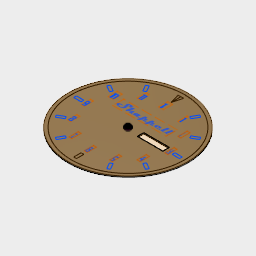
Dial (Autodesk Fusion 360 design; units mm, degrees)
Autodesk Fusion 360 part; units mm, degrees
sketch "Sketch4" plane through (0, 0, 0) normal (0, 1, 0) x (1, 0, 0)
  circle A0 centre (0, 0) radius 16.375
  dimension "d2" = 32.75
  measures "d2" diameter of A0
extrude "Extrude1" add sketch "Sketch4" along normal blind 0.35
sketch "Sketch5" plane through (0, 0.35, 0) normal (0, 1, 0) x (-1, 0, 0)
  circle A0 centre (0, 0) radius 16.375
  circle A1 centre (0, 0) radius 0.85
  line L0 (-3.45, -0.875) -> (-10.45, -0.875)
  line L1 (-10.45, -0.875) -> (-10.45, 0.875)
  line L2 (-10.45, 0.875) -> (-3.45, 0.875)
  line L3 (-3.45, 0.875) -> (-3.45, -0.875)
  dimension "d11" = 1.7
  dimension "d12" = 7
  dimension "d14" = 1.75
  dimension "d15" = 3.45
  dimension "d16" = 0.875
  measures "d11" diameter of A1
  measures "d12" distance of L0.start L0.end
  measures "d14" distance of L0.end L1.end
  measures "d15" distance of A0.centre L3
  measures "d16" distance of A0.centre L0.start
extrude "Extrude2" cut sketch "Sketch5" against normal through all contours A1 | L0 L1 L2 L3
sketch "Sketch7" plane through (0, 0.35, 0) normal (0, 1, 0) x (-1, 0, 0)
  circle A0 centre (0, 0) radius 0.85
  line L0 (-3.45, 0.875) -> (-3.45, -0.875)
  line L1 (-3.45, -0.875) -> (-10.45, -0.875)
  line L2 (-10.45, -0.875) -> (-10.45, 0.875)
  line L3 (-10.45, 0.875) -> (-3.45, 0.875)
  circle A1 centre (0, 0) radius 16.375
  line L4 (0.375, 12.5) -> (-0.375, 12.5)
  line L5 (-0.375, 12.5) -> (-0.375, 14.5)
  line L6 (-0.375, 14.5) -> (0.375, 14.5)
  line L7 (0.375, 14.5) -> (0.375, 12.5)
  circle A2 centre (0, 0) radius 15.5
  line L8 (-6.5748, 10.6378) -> (-7.5748, 12.3699)
  line L9 (-6.9252, 12.7449) -> (-5.9252, 11.0128)
  line L10 (-5.9252, 11.0128) -> (-6.5748, 10.6378)
  line L11 (-7.5748, 12.3699) -> (-6.9252, 12.7449)
  line L12 (-11.0128, 5.9252) -> (-12.7449, 6.9252)
  line L13 (-12.3699, 7.5748) -> (-10.6378, 6.5748)
  line L14 (-10.6378, 6.5748) -> (-11.0128, 5.9252)
  line L15 (-12.7449, 6.9252) -> (-12.3699, 7.5748)
  line L16 (-10.6378, -6.5748) -> (-12.3699, -7.5748)
  line L17 (-12.7449, -6.9252) -> (-11.0128, -5.9252)
  line L18 (-11.0128, -5.9252) -> (-10.6378, -6.5748)
  line L19 (-12.3699, -7.5748) -> (-12.7449, -6.9252)
  line L20 (-5.9252, -11.0128) -> (-6.9252, -12.7449)
  line L21 (-7.5748, -12.3699) -> (-6.5748, -10.6378)
  line L22 (-6.5748, -10.6378) -> (-5.9252, -11.0128)
  line L23 (-6.9252, -12.7449) -> (-7.5748, -12.3699)
  line L24 (6.5748, -10.6378) -> (7.5748, -12.3699)
  line L25 (6.9252, -12.7449) -> (5.9252, -11.0128)
  line L26 (5.9252, -11.0128) -> (6.5748, -10.6378)
  line L27 (7.5748, -12.3699) -> (6.9252, -12.7449)
  line L28 (11.0128, -5.9252) -> (12.7449, -6.9252)
  line L29 (12.3699, -7.5748) -> (10.6378, -6.5748)
  line L30 (10.6378, -6.5748) -> (11.0128, -5.9252)
  line L31 (12.7449, -6.9252) -> (12.3699, -7.5748)
  line L32 (10.6378, 6.5748) -> (12.3699, 7.5748)
  line L33 (12.7449, 6.9252) -> (11.0128, 5.9252)
  line L34 (11.0128, 5.9252) -> (10.6378, 6.5748)
  line L35 (12.3699, 7.5748) -> (12.7449, 6.9252)
  line L36 (5.9252, 11.0128) -> (6.9252, 12.7449)
  line L37 (7.5748, 12.3699) -> (6.5748, 10.6378)
  line L38 (6.5748, 10.6378) -> (5.9252, 11.0128)
  line L39 (6.9252, 12.7449) -> (7.5748, 12.3699)
  line L40 (0.75, -14.5) -> (-0.75, -14.5)
  line L41 (-0.75, -14.5) -> (0, -11.75)
  line L42 (0, -11.75) -> (0.75, -14.5)
  line L43 (0, -14.5) -> (0, -11.75)
  line L44 (-12.5, -0.375) -> (-14.5, -0.375)
  line L45 (-14.5, 0.375) -> (-12.5, 0.375)
  line L46 (-12.5, 0.375) -> (-12.5, -0.375)
  line L47 (-14.5, -0.375) -> (-14.5, 0.375)
  line L48 (12.5, 0.375) -> (14.5, 0.375)
  line L49 (14.5, -0.375) -> (12.5, -0.375)
  line L50 (12.5, -0.375) -> (12.5, 0.375)
  line L51 (14.5, 0.375) -> (14.5, -0.375)
  dimension "d20" = 0.75
  dimension "d21" = 2
  dimension "d24" = 31
  dimension "d26" = 0.375
  dimension "d31" = 2.75
  dimension "d32" = 1.5
  dimension "d33" = 0.75
  dimension "d34" = 14.5
  dimension "d35" = 14.5
  measures "d20" distance of L4.start L4.end
  measures "d21" distance of L4.start L6.end
  measures "d24" diameter of A2
  measures "d26" distance of A0.centre L4.start
  measures "d31" distance of L41.end L43.start
  measures "d32" distance of L40.start L40.end
  measures "d33" distance of A0.centre L40.end
  measures "d34" distance of A0.centre L6
  measures "d35" distance of A0.centre L40
sketch "Sketch8" plane through (0, 0.35, 0) normal (0, 1, 0) x (-1, 0, 0)
  circle A0 centre (0, 0) radius 0.85
  line L0 (-3.45, 0.875) -> (-3.45, -0.875)
  line L1 (-3.45, -0.875) -> (-10.45, -0.875)
  line L2 (-10.45, -0.875) -> (-10.45, 0.875)
  line L3 (-10.45, 0.875) -> (-3.45, 0.875)
  circle A1 centre (0, 0) radius 16.375
  line L4 (-5.4637, -8.2785) -> (-5.7091, -8.2785) construction
  line L5 (-5.7091, -8.2785) -> (-5.7091, -10.7785) construction
  line L6 (-5.7091, -10.7785) -> (-5.4637, -10.7785) construction
  line L7 (-5.4637, -10.7785) -> (-5.4637, -8.2785) construction
  line L8 (-9.0419, -4.7) -> (-9.8, -4.7) construction
  line L9 (-9.8, -4.7) -> (-9.8, -7.2) construction
  line L10 (-9.8, -7.2) -> (-9.0419, -7.2) construction
  line L11 (-9.0419, -7.2) -> (-9.0419, -4.7) construction
  line L12 (-11.1719, 1.0124) -> (-11.9349, 1.0124) construction
  line L13 (-11.9349, 1.0124) -> (-11.9349, -1.4876) construction
  line L14 (-11.9349, -1.4876) -> (-11.1719, -1.4876) construction
  line L15 (-11.1719, -1.4876) -> (-11.1719, 1.0124) construction
  line L16 (7.2613, -3.0997) -> (-7.3506, -3.0997) construction
  line L17 (-7.3506, -3.0997) -> (-7.3506, -6.0997) construction
  line L18 (-7.3506, -6.0997) -> (7.2613, -6.0997) construction
  line L19 (7.2613, -6.0997) -> (7.2613, -3.0997) construction
  line L20 (5.6532, -8.2) -> (4.9, -8.2) construction
  line L21 (4.9, -8.2) -> (4.9, -10.7) construction
  line L22 (4.9, -10.7) -> (5.6532, -10.7) construction
  line L23 (5.6532, -10.7) -> (5.6532, -8.2) construction
  line L24 (9.9968, -4.559) -> (8.654, -4.559) construction
  line L25 (8.654, -4.559) -> (8.654, -7.059) construction
  line L26 (8.654, -7.059) -> (9.9968, -7.059) construction
  line L27 (9.9968, -7.059) -> (9.9968, -4.559) construction
  line L28 (-9, 6.5) -> (-9.8447, 6.5) construction
  line L29 (-9.8447, 6.5) -> (-9.8447, 4) construction
  line L30 (-9.8447, 4) -> (-9, 4) construction
  line L31 (-9, 4) -> (-9, 6.5) construction
  line L32 (-5.2603, 10.2723) -> (-6, 10.2723) construction
  line L33 (-6, 10.2723) -> (-6, 7.7723) construction
  line L34 (-6, 7.7723) -> (-5.2603, 7.7723) construction
  line L35 (-5.2603, 7.7723) -> (-5.2603, 10.2723) construction
  line L36 (0.375, 11.567) -> (-0.3818, 11.567) construction
  line L37 (-0.3818, 11.567) -> (-0.3818, 9.067) construction
  line L38 (-0.3818, 9.067) -> (0.375, 9.067) construction
  line L39 (0.375, 9.067) -> (0.375, 11.567) construction
  line L40 (5.7526, 10.3802) -> (4.9958, 10.3802) construction
  line L41 (4.9958, 10.3802) -> (4.9958, 7.8802) construction
  line L42 (4.9958, 7.8802) -> (5.7526, 7.8802) construction
  line L43 (5.7526, 7.8802) -> (5.7526, 10.3802) construction
  line L44 (10, 6.5) -> (9.2249, 6.5) construction
  line L45 (9.2249, 6.5) -> (9.2249, 4) construction
  line L46 (9.2249, 4) -> (10, 4) construction
  line L47 (10, 4) -> (10, 6.5) construction
  line L48 (11.7568, 1) -> (11, 1) construction
  line L49 (11, 1) -> (11, -1.5) construction
  line L50 (11, -1.5) -> (11.7568, -1.5) construction
  line L51 (11.7568, -1.5) -> (11.7568, 1) construction
  line L52 (0.6011, -9.0275) -> (-0.6721, -9.0275) construction
  line L53 (-0.6721, -9.0275) -> (-0.6721, -11.5275) construction
  line L54 (-0.6721, -11.5275) -> (0.6011, -11.5275) construction
  line L55 (0.6011, -11.5275) -> (0.6011, -9.0275) construction
